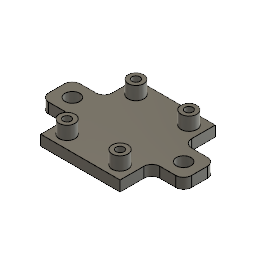
Joystick mount v1 (Autodesk Fusion 360 design; units mm, degrees)
Autodesk Fusion 360 part; units mm, degrees
note: some values were not read from the file. Set by a fixed rule: which sketch regions a step uses.
sketch "Sketch1" plane through (0, 0, 0) normal (0, 1, 0) x (1, 0, 0)
  line L0 (10, 13) -> (-10, 13) construction
  line L1 (-10, 13) -> (-10, -13) construction
  line L2 (-10, -13) -> (10, -13) construction
  line L3 (10, -13) -> (10, 13) construction
  line L4 (10, 13) -> (-10, -13) construction
  line L5 (-10, 13) -> (10, -13) construction
  circle A0 centre (10, 13) radius 1.5
  line L6 (0, 0) -> (0, 6) construction
  line L7 (0, 0) -> (-6, 0) construction
  line L8 (2.5, 0) -> (20, 0)
  circle A1 centre (10, -13) radius 1.5
  line L9 (0, -20) -> (0, -2.5)
  circle A2 centre (-10, 13) radius 1.5
  circle A3 centre (-10, -13) radius 1.5
  circle A4 centre (-10, -13) radius 3
  circle A5 centre (-10, 13) radius 3
  circle A6 centre (10, -13) radius 3
  circle A7 centre (10, 13) radius 3
  line L10 (15, -18) -> (-15, -18)
  line L11 (-15, -18) -> (-15, 18)
  line L12 (-15, 18) -> (15, 18)
  line L13 (15, 18) -> (15, -18)
  line L14 (15, -18) -> (-15, 18) construction
  line L15 (-15, -18) -> (15, 18) construction
  line L16 (15, -6) -> (27, -6)
  line L17 (27, -6) -> (27, 6)
  line L18 (27, 6) -> (15, 6)
  line L19 (15, 6) -> (15, -6)
  line L20 (15, -6) -> (27, 6) construction
  line L21 (27, -6) -> (15, 6) construction
  circle A8 centre (21, 0) radius 2.75
  circle A9 centre (-21, 0) radius 2.75
  line L22 (-15, -6) -> (-27, -6)
  line L23 (-27, -6) -> (-27, 6)
  line L24 (-27, 6) -> (-15, 6)
  point P0 (21, 0)
  dimension "d1" = 3
  dimension "d2" = 1.5
  dimension "d3" = 26
  dimension "d4" = 20
  dimension "d5" = 5
  dimension "d6" = 5
  dimension "d7" = 12
  dimension "d8" = 12
  dimension "d9" = 5.5
  constraint perpendicular L0 L1
  constraint parallel L0 L2
  constraint parallel L1 L3
  constraint horizontal L0
  constraint coincident L4 L6.start
  constraint coincident L5 L6.start
  constraint coincident L6.start L7.start
  constraint coincident L0.start L3.end
  constraint vertical L6
  constraint perpendicular L6 L7
  constraint symmetric A0 L8 A1
  constraint symmetric A0 L9 A2
  constraint symmetric A1 L9 A3
  constraint concentric A3 A4
  constraint symmetric L8 A4 A5
  constraint symmetric L9 A4 A6
  constraint symmetric L9 A5 A7
  constraint perpendicular L10 L11
  constraint parallel L10 L12
  constraint parallel L11 L13
  constraint horizontal L10
  constraint coincident L14 L6.start
  constraint coincident L15 L6.start
  constraint perpendicular L16 L17
  constraint parallel L16 L18
  constraint parallel L17 L19
  constraint horizontal L16
  constraint coincident L13 L16.start
  constraint coincident L20 P0
  constraint coincident L21 P0
  constraint coincident L8 P0
  constraint coincident P0 A8.centre
  constraint symmetric L9 L16.start L22.start
  constraint symmetric L9 L16.end L22.end
  constraint symmetric L9 L17.end L23.end
  constraint symmetric L9 L18.end L24.end
  constraint symmetric L9 A8 A9
  measures "d1" diameter of A3
  measures "d2" distance of A1 A6
  measures "d3" distance of L2.end L0.start
  measures "d4" distance of L2.end L1.end
  measures "d5" distance of L2.end L10
  measures "d6" distance of L2.end L13
  measures "d7" distance of L17 L19
  measures "d8" distance of L16 L18
  measures "d9" diameter of A8
extrude "Extrude1" add sketch "Sketch1" against normal blind 4 contours A0 | A1 | A2 | A3 | A4 | A5 | A6 | A7 | L10 L11 L12 L13 L19 | L13 L16 L17 L18 L19 | L11 L22 L23 L24
extrude "Extrude2" add sketch "Sketch1" along normal blind 5 contours A4 | A5 | A6 | A7
extrude "Extrude3" cut sketch "Sketch1" against normal blind 3 contours A0 | A1 | A2 | A3
fillet "Fillet1" radius 3 8 edges at (-27, -2, -6) (-27, -2, 6) (27, -2, -6) (27, -2, 6) (15, -2, -6) (15, -2, 6) (-15, -2, 6) (-15, -2, -6)
